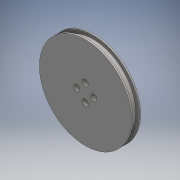
# Autodesk Inventor part: LargeWheel
Saved by Autodesk Inventor 2016 (Build 200138000, 138)
## iProperties
Created: 2016-03-28
Part Number: LargeWheel
Material: Generic
Document SubType Name: Modeling
Designer: mkepler
Density: 1 g/cm^3
Appearance: Default
Author: mkepler
Autodesk Inventor part; units mm, degrees
ref_plane "YZ Plane" through (0, 0, 0) normal (1, 0, 0) x (0, 1, 0)
ref_plane "XZ Plane" through (0, 0, 0) normal (0, 1, 0) x (-1, 0, 0)
ref_plane "XY Plane" through (0, 0, 0) normal (0, 0, 1) x (1, 0, 0)
sketch "Sketch1" plane through (0, 0, 0) normal (0, 1, 0) x (-1, 0, 0)
  circle A0 centre (0, 0) radius 32.5
  dimension "d0" = 65
  constraints: 1 centre point, 1 coincident
  measures "d0" diameter of A0
extrude "Extrusion1" add sketch "Sketch1" along normal blind 1
sketch "Sketch2" plane through (0, 1, 0) normal (0, 1, 0) x (1, 0, 0)
  circle A0 centre (0, 0) radius 30
  dimension "d3" = 60
  constraints: 1 centre point, 1 coincident
  measures "d3" diameter of A0
extrude "Extrusion2" add sketch "Sketch2" along normal blind 4.5
sketch "Sketch3" plane through (0, 5.5, 0) normal (0, 1, 0) x (1, 0, 0)
  circle A0 centre (0, 0) radius 32.5
  dimension "d6" = 65
  constraints: 1 centre point, 1 coincident
  measures "d6" diameter of A0
extrude "Extrusion3" add sketch "Sketch3" along normal blind 1
sketch "Sketch4" plane through (0, 6.5, 0) normal (0, 1, 0) x (1, 0, 0)
  circle A0 centre (0, 0) radius 9.75
  dimension "d9" = 19.5
  constraints: 1 centre point, 1 coincident
  measures "d9" diameter of A0
extrude "Extrusion4" cut sketch "Sketch4" against normal blind 1.5
sketch "Sketch5" plane through (0, 5, 0) normal (0, 1, 0) x (1, 0, 0)
  circle A0 centre (0, 6) radius 2.15
  circle A1 centre (0, -6) radius 2.15
  circle A2 centre (-6, 0) radius 2.15
  circle A3 centre (6, 0) radius 2.15
  point P0 (0, 0)
  dimension "d12" = 4.3
  dimension "d13" = 6
  dimension "d14" = 4.3
  dimension "d15" = 12
  dimension "d16" = 4.3
  dimension "d17" = 6
  dimension "d18" = 4.3
  dimension "d19" = 12
  constraints: 4 centre point
  measures "d12" diameter of A0
  measures "d13" distance of A0.centre point (0, 0)
  measures "d14" diameter of A1
  measures "d15" distance of A1.centre A0.centre
  measures "d16" diameter of A2
  measures "d17" distance of A2.centre point (0, 0)
  measures "d18" diameter of A3
  measures "d19" distance of A3.centre A2.centre
hole "Hole1" at (0, 5, -6) at (6, 5, 0) at (0, 5, 6) at (-6, 5, 0) direction (0, -1, 0) diameter 4.3 end through all
body "Solid1"
